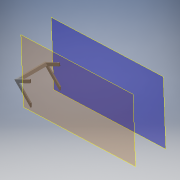
# Autodesk Inventor part: RearCrumple
Saved by Autodesk Inventor 2018 (Build 220112000, 112)
## iProperties
Created: 2018-05-15
Part Number: RearCrumple
Material: Generic
Document SubType Name: Modeling
Designer: andrecheke21
Density: 1 g/cm^3
Appearance: Default
Author: andrecheke21
Autodesk Inventor part; units mm, degrees
ref_plane "YZ Plane" through (0, 0, 0) normal (1, 0, 0) x (0, 1, 0)
ref_plane "XZ Plane" through (0, 0, 0) normal (0, 1, 0) x (-1, 0, 0)
ref_plane "XY Plane" through (0, 0, 0) normal (0, 0, 1) x (1, 0, 0)
ref_plane "Work Plane1" through (1143.7783, 851.9673, -406.3915) normal (0, 0, -1) x (-0.8080578, -0.5891032, 0)
sketch "Sketch1" plane through (1143.7783, 851.9673, -406.3915) normal (0, 0, -1) x (-0.8080578, -0.5891032, 0)
  line L0 (1269.8194, 209.303) -> (1593.8019, 73.5805)
  line L1 (1593.8019, 73.5805) -> (1269.8194, -281.049)
  line L2 (1259.4205, 173.4665) -> (1567.246, 44.5125)
  line L3 (1511.4503, 67.8864) -> (1259.4205, -207.9841)
  line L4 (1259.4205, 213.6593) -> (1259.4205, 173.4665)
  line L5 (1259.4205, -207.9841) -> (1269.8194, -281.049)
  point P0 (1426.1356, -14.6355)
  constraints: 12 end point, 3 point on line, 1 parallel, 1 vertical
extrude "Extrusion1" add sketch "Sketch1" against normal blind 25.4
ref_plane "Work Plane3" through (1143.7783, 851.9673, -406.3915) normal (0, 0, -1) x (-0.8080578, -0.5891032, 0)
sketch "Sketch3" plane through (1143.7783, 851.9673, -406.3915) normal (0, 0, -1) x (-0.8080578, -0.5891032, 0)
  line L0 (1264.3348, 241.5423) -> (1610.7303, 93.3818)
  line L1 (1511.4503, 67.8864) -> (1567.246, 44.5125) projected
  line L2 (1610.7303, 93.3818) -> (1567.246, 44.5125)
  line L3 (1567.246, 44.5125) -> (1264.3348, 174.0739)
  line L4 (1264.3348, 174.0739) -> (1264.3348, 241.5423)
  point P0 (1426.1356, -14.6355)
  constraints: 8 end point, 1 parallel, 1 vertical
extrude "Extrusion3" add sketch "Sketch3" against normal blind 25.4
ref_plane "Work Plane4" through (1129.2131, 527.0149, 254.0085) normal (0, 0, 1) x (0.8080578, 0.5891032, 0)
sketch "Sketch4" plane through (1129.2131, 527.0149, 254.0085) normal (0, 0, 1) x (0.8080578, 0.5891032, 0)
  line L0 (-1061.1348, 428.0739) -> (-1061.1348, 495.5423) projected
  line L1 (-1061.1348, 495.5423) -> (-1407.5303, 347.3818) projected
  line L2 (-1061.1348, 495.5423) -> (-1407.5303, 347.3818)
  line L3 (-1364.046, 298.5125) -> (-1066.6194, -27.049) projected
  line L4 (-1407.5303, 347.3818) -> (-1066.6194, -27.049)
  line L5 (-1066.6194, -27.049) -> (-1066.6194, 56.4973)
  line L6 (-1308.2503, 321.8864) -> (-1364.046, 298.5125) projected
  line L7 (-1066.6194, 56.4973) -> (-1308.2503, 321.8864)
  line L8 (-1364.046, 298.5125) -> (-1061.1348, 428.0739) projected
  line L9 (-1308.2503, 321.8864) -> (-1061.1348, 428.0739)
  line L10 (-1061.1348, 428.0739) -> (-1061.1348, 495.5423)
  line L11 (-1407.5303, 347.3818) -> (-1364.046, 298.5125) projected
  line L12 (-1407.5303, 347.3818) -> (-1343.0061, 374.9801)
  line L13 (-1308.2503, 321.8864) -> (-1364.046, 298.5125)
  point P0 (-1222.9356, 239.3645)
  point P1 (-1364.046, 298.5125)
  point P2 (-1293.9365, 306.2186)
  constraints: 16 end point, 2 parallel, 1 collinear, 1 point on line, 1 vertical, 1 other
extrude "Extrusion4" add sketch "Sketch4" against normal blind 25.4 contours L8 L4 L1 L0 | L9 L6 L4 L8 | L7 L5 L4 L6
sketch "Sketch5" plane through (1143.7783, 851.9673, -380.9915) normal (0, 0, 1) x (0.8080578, 0.5891032, 0)
  line L0 (-1567.246, 44.5125) -> (-1264.3348, 174.0739) projected
  line L1 (-1514.0603, 67.2611) -> (-1559.35, 115.3583)
  line L2 (-1264.3348, 241.5423) -> (-1610.7303, 93.3818) projected
  line L3 (-1610.7303, 93.3818) -> (-1559.35, 38.8164)
  line L4 (-1559.35, 38.8164) -> (-1521.1481, 74.7883)
  point P0 (-1426.1356, -14.6355)
  point P1 (-1264.3348, 174.0739)
  point P2 (-1584.1346, -28.1729)
  constraints: 6 end point, 2 point on line, 1 parallel, 1 perpendicular, 2 other
extrude "Extrusion5" add sketch "Sketch5" along normal blind 635 contours L3 L2 L1 L4 L0 | L0 L4 L3
body "Solid1"
